# Autodesk Inventor part: m3_nut_locking
Saved by Autodesk Inventor 2021 (Build 250183000, 183)
## iProperties
Created: 2021-03-15
Part Number: m3_nut_locking
Material: Stainless Steel
Document SubType Name: Modeling
Designer: Tomasz Lisowski
Density: 8 g/cm^3
Appearance: Semi-Polished
Author: Tomasz Lisowski
Autodesk Inventor part; units mm, degrees
ref_plane "YZ Plane" through (0, 0, 0) normal (1, 0, 0) x (0, 1, 0)
ref_plane "XZ Plane" through (0, 0, 0) normal (0, 1, 0) x (-1, 0, 0)
ref_plane "XY Plane" through (0, 0, 0) normal (0, 0, 1) x (1, 0, 0)
sketch "Sketch1" plane through (0, 0, 0) normal (0, 1, 0) x (-1, 0, 0)
  line L0 (0, -3.1177) -> (-2.7, -1.5588)
  line L1 (-2.7, -1.5588) -> (-2.7, 1.5588)
  line L2 (-2.7, 1.5588) -> (0, 3.1177)
  line L3 (0, 3.1177) -> (2.7, 1.5588)
  line L4 (2.7, 1.5588) -> (2.7, -1.5588)
  line L5 (2.7, -1.5588) -> (0, -3.1177)
  circle A0 centre (0, 0) radius 1.5
  dimension "d0" = 5.4
  dimension "d1" = 3
  constraints: 12 end point, 2 coincident, 1 centre point, 1 vertical alignment, 13 other
  measures "d0" distance between parallel lines of L1 L4
  measures "d1" diameter of A0
extrude "Extrusion1" add sketch "Sketch1" along normal blind 2.4
sketch "Sketch2" plane through (0, 2.4, 0) normal (0, 1, 0) x (1, 0, 0)
  circle A0 centre (0, 0) radius 2.7
  line L0 (2.7, -1.5588) -> (2.7, 1.5588) projected
  line L1 (-2.7, 1.5588) -> (-2.7, -1.5588) projected
  circle A1 centre (0, 0) radius 1.5 projected
  dimension "d4" = 5.4
  dimension "d5" = 5.4
  constraints: 1 centre point, 1 coincident
  measures "d4" distance between parallel lines of L0 L1
  measures "d5" diameter of A0
extrude "Extrusion2" add sketch "Sketch2" along normal blind 1.4
fillet "Fillet1" radius 0.4 1 edges at (-2.7, 3.8, 0)
equation "\"d5\" = d4"
body "Solid1"
